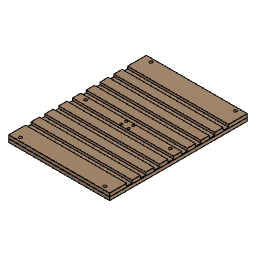
X platform (Autodesk Fusion 360 design; units mm, degrees)
Autodesk Fusion 360 part; units mm, degrees
sketch "Bottom" plane through (0, 0, 0) normal (0, 0, 1) x (1, 0, 0)
  line L0 (275, 375) -> (-275, 375)
  line L1 (-275, 375) -> (-275, -375)
  line L2 (-275, -375) -> (275, -375)
  line L3 (275, -375) -> (275, 375)
  line L4 (275, 375) -> (-275, -375) construction
  line L5 (-275, 375) -> (275, -375) construction
  line L6 (155, 375) -> (155, -375) construction
  line L7 (-155, 375) -> (-155, -375) construction
  line L8 (-155, 349.39) -> (-140, 349.39) construction
  line L9 (-140, 349.39) -> (-140, -349.39) construction
  line L10 (-140, -349.39) -> (-170, -349.39) construction
  line L11 (-170, -349.39) -> (-170, 349.39) construction
  line L12 (-170, 349.39) -> (-155, 349.39) construction
  line L13 (155, 350.2785) -> (170, 350.2785) construction
  line L14 (170, 350.2785) -> (170, -350.2785) construction
  line L15 (170, -350.2785) -> (140, -350.2785) construction
  line L16 (140, -350.2785) -> (140, 350.2785) construction
  line L17 (140, 350.2785) -> (155, 350.2785) construction
  line L18 (-170, 0) -> (170, 0) construction
  line L19 (-170, 300) -> (170, 300) construction
  line L20 (-170, 150) -> (170, 150) construction
  line L21 (-170, -150) -> (170, -150) construction
  line L22 (-170, -300) -> (170, -300) construction
  circle A0 centre (-170, -300) radius 3
  circle A1 centre (-140, -300) radius 3
  circle A2 centre (140, -300) radius 3
  circle A3 centre (170, -300) radius 3
  circle A4 centre (-170, -150) radius 3
  circle A5 centre (-140, -150) radius 3
  circle A6 centre (140, -150) radius 3
  circle A7 centre (170, -150) radius 3
  circle A8 centre (-170, 0) radius 3
  circle A9 centre (-140, 0) radius 3
  circle A10 centre (140, 0) radius 3
  circle A11 centre (170, 0) radius 3
  circle A12 centre (-170, 150) radius 3
  circle A13 centre (-140, 150) radius 3
  circle A14 centre (140, 150) radius 3
  circle A15 centre (170, 150) radius 3
  circle A16 centre (-170, 300) radius 3
  circle A17 centre (-140, 300) radius 3
  circle A18 centre (140, 300) radius 3
  circle A19 centre (170, 300) radius 3
  line L23 (-18.5, 7) -> (21.5, 7) construction
  line L24 (21.5, 7) -> (21.5, -17) construction
  line L25 (21.5, -17) -> (-18.5, -17) construction
  line L26 (-18.5, -17) -> (-18.5, 7) construction
  circle A20 centre (-18.5, 7) radius 3
  circle A21 centre (21.5, 7) radius 3
  circle A22 centre (21.5, -17) radius 3
  circle A23 centre (-18.5, -17) radius 3
  circle A24 centre (-230, 355) radius 3.5
  circle A25 centre (-230, 355) radius 7.95
  circle A26 centre (230, 355) radius 3.5
  circle A27 centre (230, 355) radius 7.95
  circle A28 centre (230, -355) radius 3.5
  circle A29 centre (230, -355) radius 7.95
  circle A30 centre (-230, -355) radius 3.5
  circle A31 centre (-230, -355) radius 7.95
  circle A32 centre (-170, 300) radius 6.35
  circle A33 centre (-140, 300) radius 6.35
  circle A34 centre (-170, 150) radius 6.35
  circle A35 centre (-140, 150) radius 6.35
  circle A36 centre (-170, 0) radius 6.35
  circle A37 centre (-140, 0) radius 6.35
  circle A38 centre (-170, -150) radius 6.35
  circle A39 centre (-140, -150) radius 6.35
  circle A40 centre (-170, -300) radius 6.35
  circle A41 centre (-140, -300) radius 6.35
  circle A42 centre (140, -300) radius 6.35
  circle A43 centre (170, -300) radius 6.35
  circle A44 centre (140, -150) radius 6.35
  circle A45 centre (170, -150) radius 6.35
  circle A46 centre (140, 0) radius 6.35
  circle A47 centre (170, 0) radius 6.35
  circle A48 centre (140, 150) radius 6.35
  circle A49 centre (170, 150) radius 6.35
  circle A50 centre (140, 300) radius 6.35
  circle A51 centre (170, 300) radius 6.35
  circle A52 centre (-18.5, 7) radius 6.35
  circle A53 centre (21.5, 7) radius 6.35
  circle A54 centre (-18.5, -17) radius 6.35
  circle A55 centre (21.5, -17) radius 6.35
  line L27 (230, -355) -> (230, 355) construction
  line L28 (-230, 355) -> (-230, -355) construction
  circle A56 centre (230, 0) radius 3.5
  circle A57 centre (230, 0) radius 7.95
  circle A58 centre (-230, 0) radius 3.5
  circle A59 centre (-230, 0) radius 7.95
  dimension "d1" = 550
  dimension "d2" = 750
  dimension "d3" = 120
  dimension "d4" = 310
  dimension "d5" = 120
  dimension "d6" = 30
  dimension "d7" = 30
  dimension "d9" = 150
  dimension "d10" = 150
  dimension "d11" = 150
  dimension "d12" = 150
  dimension "d13" = 6
  dimension "d14" = 6
  dimension "d15" = 6
  dimension "d16" = 6
  dimension "d17" = 6
  dimension "d18" = 6
  dimension "d19" = 6
  dimension "d20" = 6
  dimension "d21" = 6
  dimension "d22" = 6
  dimension "d23" = 6
  dimension "d24" = 6
  dimension "d25" = 6
  dimension "d26" = 6
  dimension "d27" = 6
  dimension "d28" = 6
  dimension "d29" = 6
  dimension "d30" = 6
  dimension "d31" = 6
  dimension "d32" = 6
  dimension "d33" = 75
  dimension "d36" = 24
  dimension "d37" = 368
  dimension "d38" = 358
  dimension "d39" = 253.5
  dimension "d40" = 256.5
  dimension "d41" = 40
  dimension "d42" = 6
  dimension "d43" = 6
  dimension "d44" = 6
  dimension "d45" = 6
  dimension "d46" = 7
  dimension "d47" = 15.9
  dimension "d48" = 20
  dimension "d49" = 45
  dimension "d50" = 7
  dimension "d51" = 15.9
  dimension "d52" = 45
  dimension "d53" = 20
  dimension "d54" = 7
  dimension "d55" = 15.9
  dimension "d56" = 45
  dimension "d57" = 20
  dimension "d58" = 7
  dimension "d59" = 15.9
  dimension "d60" = 20
  dimension "d61" = 45
  dimension "d74" = 12.7
  dimension "d75" = 12.7
  dimension "d76" = 12.7
  dimension "d77" = 12.7
  dimension "d78" = 12.7
  dimension "d79" = 12.7
  dimension "d80" = 12.7
  dimension "d81" = 12.7
  dimension "d82" = 12.7
  dimension "d83" = 12.7
  dimension "d84" = 12.7
  dimension "d85" = 12.7
  dimension "d86" = 12.7
  dimension "d87" = 12.7
  dimension "d88" = 12.7
  dimension "d89" = 12.7
  dimension "d90" = 12.7
  dimension "d91" = 12.7
  dimension "d92" = 12.7
  dimension "d93" = 12.7
  dimension "d122" = 12.7
  dimension "d123" = 12.7
  dimension "d124" = 12.7
  dimension "d125" = 12.7
  dimension "d167" = 7
  dimension "d168" = 15.9
  dimension "d169" = 7
  dimension "d170" = 15.9
  constraint perpendicular L0 L1
  constraint parallel L0 L2
  constraint parallel L1 L3
  constraint horizontal L0
  constraint coincident L4 origin
  constraint coincident L5 origin
  constraint coincident L0 L6.start
  constraint perpendicular L0 L6
  constraint coincident L0 L7.start
  constraint coincident L2 L7.end
  constraint perpendicular L2 L7
  constraint coincident L7 L8.start
  constraint perpendicular L7 L8
  constraint perpendicular L8 L9
  constraint perpendicular L7 L10
  constraint perpendicular L10 L11
  constraint collinear L8 L12
  constraint equal L8 L12
  constraint coincident L6 L13.start
  constraint perpendicular L6 L13
  constraint perpendicular L13 L14
  constraint perpendicular L6 L15
  constraint perpendicular L15 L16
  constraint perpendicular L6 L17
  constraint equal L13 L17
  constraint midpoint L11 L18.start
  constraint midpoint L14 L18.end
  constraint coincident L11 L19.start
  constraint coincident L14 L19.end
  constraint perpendicular L14 L19
  constraint perpendicular L9 L18
  constraint coincident L11 L20.start
  constraint coincident L14 L20.end
  constraint perpendicular L14 L20
  constraint coincident L11 L21.start
  constraint coincident L14 L21.end
  constraint perpendicular L14 L21
  constraint coincident L11 L22.start
  constraint coincident L14 L22.end
  constraint perpendicular L14 L22
  constraint coincident L22.start A0.centre
  constraint coincident L9 A1.centre
  constraint coincident L22 A1.centre
  constraint coincident L16 A2.centre
  constraint coincident L22 A2.centre
  constraint coincident L22.end A3.centre
  constraint coincident L21.start A4.centre
  constraint coincident L9 A5.centre
  constraint coincident L21 A5.centre
  constraint coincident L16 A6.centre
  constraint coincident L21 A6.centre
  constraint coincident L21.end A7.centre
  constraint coincident L18.start A8.centre
  constraint midpoint L9 A9.centre
  constraint midpoint L16 A10.centre
  constraint coincident L18.end A11.centre
  constraint coincident L20.start A12.centre
  constraint coincident L9 A13.centre
  constraint coincident L20 A13.centre
  constraint coincident L16 A14.centre
  constraint coincident L20 A14.centre
  constraint coincident L20.end A15.centre
  constraint coincident L19.start A16.centre
  constraint coincident L19 A17.centre
  constraint coincident L9 A17.centre
  constraint coincident L16 A18.centre
  constraint coincident L19 A18.centre
  constraint coincident L19.end A19.centre
  constraint horizontal L23
  constraint vertical L24
  constraint horizontal L25
  constraint vertical L26
  constraint coincident L23.start L26.end
  constraint coincident L23.end L24.start
  constraint coincident L24.end L25.start
  constraint coincident L25.end L26.start
  constraint concentric A24 A25
  constraint concentric A26 A27
  constraint concentric A28 A29
  constraint concentric A30 A31
  constraint concentric A16 A32
  constraint concentric A17 A33
  constraint concentric A12 A34
  constraint concentric A13 A35
  constraint concentric A8 A36
  constraint concentric A9 A37
  constraint concentric A4 A38
  constraint concentric A5 A39
  constraint concentric A0 A40
  constraint concentric A1 A41
  constraint concentric A2 A42
  constraint concentric A3 A43
  constraint concentric A6 A44
  constraint concentric A7 A45
  constraint concentric A10 A46
  constraint concentric A11 A47
  constraint concentric A14 A48
  constraint concentric A15 A49
  constraint concentric A18 A50
  constraint concentric A19 A51
  constraint concentric A20 A52
  constraint concentric A21 A53
  constraint concentric A23 A54
  constraint concentric A22 A55
  constraint coincident A28.centre A29.centre
  constraint coincident A26.centre A27.centre
  constraint coincident A24.centre A25.centre
  constraint coincident A30.centre A31.centre
  constraint midpoint L27 A56.centre
  constraint concentric A56 A57
  constraint midpoint L28 A58.centre
  constraint concentric A58 A59
  measures "d1" distance of L1.end L2.end
  measures "d2" distance of L0.end L1.end
  measures "d3" distance of L3 L6
  measures "d4" distance of L6 L7
  measures "d5" distance of L1 L7
  measures "d6" distance of L9 L11
  measures "d7" distance of L14 L16
  measures "d9" distance of L18 L20
  measures "d10" distance of L19 L20
  measures "d11" distance of L18 L21
  measures "d12" distance of L21 L22
  measures "d13" diameter of A0
  measures "d14" diameter of A1
  measures "d15" diameter of A2
  measures "d16" diameter of A3
  measures "d17" diameter of A4
  measures "d18" diameter of A5
  measures "d19" diameter of A6
  measures "d20" diameter of A7
  measures "d21" diameter of A8
  measures "d22" diameter of A9
  measures "d23" diameter of A10
  measures "d24" diameter of A11
  measures "d25" diameter of A12
  measures "d26" diameter of A13
  measures "d27" diameter of A14
  measures "d28" diameter of A15
  measures "d29" diameter of A16
  measures "d30" diameter of A17
  measures "d31" diameter of A18
  measures "d32" diameter of A19
  measures "d33" distance of L0 L19
  measures "d36" distance of L23.start L25.end
  measures "d37" distance of L0 L23
  measures "d38" distance of L2 L25
  measures "d39" distance of L3 L24
  measures "d40" distance of L1 L26
  measures "d41" distance of L24 L26
  measures "d42" diameter of A20
  measures "d43" diameter of A21
  measures "d44" diameter of A22
  measures "d45" diameter of A23
  measures "d46" diameter of A24
  measures "d47" diameter of A25
  measures "d48" distance of L0 A24.centre
  measures "d49" distance of L1 A24.centre
  measures "d50" diameter of A26
  measures "d51" diameter of A27
  measures "d52" distance of L3 A26.centre
  measures "d53" distance of L0 A26.centre
  measures "d54" diameter of A28
  measures "d55" diameter of A29
  measures "d56" distance of L3 A28.centre
  measures "d57" distance of L2 A28.centre
  measures "d58" diameter of A30
  measures "d59" diameter of A31
  measures "d60" distance of L2 A30.centre
  measures "d61" distance of L1 A30.centre
  measures "d74" diameter of A32
  measures "d75" diameter of A33
  measures "d76" diameter of A34
  measures "d77" diameter of A35
  measures "d78" diameter of A36
  measures "d79" diameter of A37
  measures "d80" diameter of A38
  measures "d81" diameter of A39
  measures "d82" diameter of A40
  measures "d83" diameter of A41
  measures "d84" diameter of A42
  measures "d85" diameter of A43
  measures "d86" diameter of A44
  measures "d87" diameter of A45
  measures "d88" diameter of A46
  measures "d89" diameter of A47
  measures "d90" diameter of A48
  measures "d91" diameter of A49
  measures "d92" diameter of A50
  measures "d93" diameter of A51
  measures "d122" diameter of A52
  measures "d123" diameter of A53
  measures "d124" diameter of A54 L0.start
  measures "d125" diameter of A55
  measures "d167" diameter of A56
  measures "d168" diameter of A57
  measures "d169" diameter of A58
  measures "d170" diameter of A59
extrude "Extrude24" add sketch "Bottom" against normal blind 18 contours L0 L1 L2 L3 | A25 | A27 | A29 | A31 | A32 | A33 | A34 | A35 | A36 | A37 | A38 | A39 | A40 | A41 | A42 | A43 | A44 | A45 | A46 | A47 | A48 | A49 | A50 | A51 | A52 | A53 | A54 | A55 | A57 | A59 makes body 1
extrude "Extrude27" cut sketch "Bottom" against normal through all from surface at -9 contours A25 | A27 | A29 | A31 | A57 | A59 bodies 1
extrude "Extrude28" cut sketch "Bottom" against normal blind 8 contours A32 | A33 | A34 | A35 | A36 | A37 | A38 | A39 | A40 | A41 | A42 | A43 | A44 | A45 | A46 | A47 | A48 | A49 | A50 | A51 bodies 1
fillet "Fillet1" radius 0.5 12 edges at (-275, 0, 0) (-275, 0, -18) (0, -375, 0) (0, -375, -18) (275, 0, 0) (275, 0, -18) (0, 375, 0) (0, 375, -18) (-275, 375, -9) (-275, -375, -9) (275, -375, -9) (275, 375, -9) on bodies 1
extrude "Extrude25" add sketch "Bottom" along normal blind 8 separate body contours A25 | A27 | A29 | A31 | A57 | A59 makes body 2 at (237.7042, -353.0383, 5.3333) makes body 3 at (-222.2958, 356.9617, 5.3333) makes body 4 at (-222.2958, -353.0383, 5.3333) makes body 5 at (237.7042, 356.9617, 5.3333) makes body 6 at (-222.0599, -0.3963, 5.3333) makes body 7 at (237.9401, -0.3963, 5.3333)
extrude "Extrude26" add sketch "Bottom" along normal blind 18 contours L0 L1 L2 L3 | A0 | A1 | A2 | A3 | A4 | A5 | A6 | A7 | A8 | A9 | A10 | A11 | A12 | A13 | A14 | A15 | A16 | A17 | A18 | A19 | A32 | A33 | A34 | A35 | A36 | A37 | A38 | A39 | A40 | A41 | A42 | A43 | A44 | A45 | A46 | A47 | A48 | A49 | A50 | A51 bodies 6 3 7 2 5 4
extrude "Extrude29" cut sketch "Bottom" along normal blind 8 contours A0 | A1 | A2 | A3 | A4 | A5 | A6 | A7 | A8 | A9 | A10 | A11 | A12 | A13 | A14 | A15 | A16 | A17 | A18 | A19 | A20 | A21 | A22 | A23 | A32 | A33 | A34 | A35 | A36 | A37 | A38 | A39 | A40 | A41 | A42 | A43 | A44 | A45 | A46 | A47 | A48 | A49 | A50 | A51 | A52 | A53 | A54 | A55 bodies 6
fillet "Fillet3" radius 0.5 12 edges at (0, 375, 18) (0, 375, 0) (-275, 375, 9) (-275, 0, 18) (-275, 0, 0) (-275, -375, 9) (0, -375, 18) (0, -375, 0) (275, 375, 9) (275, 0, 18) (275, 0, 0) (275, -375, 9) on bodies 6
sketch "Side" plane through (275, 0, 0) normal (1, 0, 0) x (0, 1, 0)
  line L0 (-375, 0) -> (375, 0)
  line L1 (375, 0) -> (375, 25)
  line L2 (375, 25) -> (-375, 25)
  line L3 (-375, 25) -> (-375, 0)
  line L4 (-391.2499, 11.5) -> (399.4526, 11.5) construction
  line L5 (399.4526, 11.5) -> (389.4526, 11.5) construction
  line L6 (-27.5, 18) -> (-57.5, 18)
  line L7 (-57.5, 18) -> (-57.5, 5)
  line L8 (-57.5, 5) -> (-27.5, 5)
  line L9 (-27.5, 5) -> (-27.5, 18)
  line L10 (-27.5, 18) -> (-57.5, 5) construction
  line L11 (-57.5, 18) -> (-27.5, 5) construction
  line L12 (-102.5, 18) -> (-132.5, 18)
  line L13 (-132.5, 18) -> (-132.5, 5)
  line L14 (-132.5, 5) -> (-102.5, 5)
  line L15 (-102.5, 5) -> (-102.5, 18)
  line L16 (-102.5, 18) -> (-132.5, 5) construction
  line L17 (-132.5, 18) -> (-102.5, 5) construction
  line L18 (47.5, 18) -> (17.5, 18)
  line L19 (17.5, 18) -> (17.5, 5)
  line L20 (17.5, 5) -> (47.5, 5)
  line L21 (47.5, 5) -> (47.5, 18)
  line L22 (47.5, 18) -> (17.5, 5) construction
  line L23 (17.5, 18) -> (47.5, 5) construction
  line L24 (122.5, 18) -> (92.5, 18)
  line L25 (92.5, 18) -> (92.5, 5)
  line L26 (92.5, 5) -> (122.5, 5)
  line L27 (122.5, 5) -> (122.5, 18)
  line L28 (122.5, 18) -> (92.5, 5) construction
  line L29 (92.5, 18) -> (122.5, 5) construction
  line L30 (197.5, 18) -> (167.5, 18)
  line L31 (167.5, 18) -> (167.5, 5)
  line L32 (167.5, 5) -> (197.5, 5)
  line L33 (197.5, 5) -> (197.5, 18)
  line L34 (197.5, 18) -> (167.5, 5) construction
  line L35 (167.5, 18) -> (197.5, 5) construction
  line L36 (-177.5, 18) -> (-207.5, 18)
  line L37 (-207.5, 18) -> (-207.5, 5)
  line L38 (-207.5, 5) -> (-177.5, 5)
  line L39 (-177.5, 5) -> (-177.5, 18)
  line L40 (-177.5, 18) -> (-207.5, 5) construction
  line L41 (-207.5, 18) -> (-177.5, 5) construction
  line L42 (272.5, 18) -> (242.5, 18)
  line L43 (242.5, 18) -> (242.5, 5)
  line L44 (242.5, 5) -> (272.5, 5)
  line L45 (272.5, 5) -> (272.5, 18)
  line L46 (272.5, 18) -> (242.5, 5) construction
  line L47 (242.5, 18) -> (272.5, 5) construction
  line L48 (-252.5, 18) -> (-282.5, 18)
  line L49 (-282.5, 18) -> (-282.5, 5)
  line L50 (-282.5, 5) -> (-252.5, 5)
  line L51 (-252.5, 5) -> (-252.5, 18)
  line L52 (-252.5, 18) -> (-282.5, 5) construction
  line L53 (-282.5, 18) -> (-252.5, 5) construction
  line L54 (-375, 0) -> (375, 0)
  line L55 (-374.5, 17.5) -> (-374.5, 0.5)
  line L56 (-374.5, 0.5) -> (374.5, 0.5)
  line L57 (374.5, 0.5) -> (374.5, 17.5)
  line L58 (374.5, 17.5) -> (-374.5, 17.5)
  point P0 (-42.5, 11.5)
  point P1 (-117.5, 11.5)
  point P2 (32.5, 11.5)
  point P3 (107.5, 11.5)
  point P4 (182.5, 11.5)
  point P5 (-192.5, 11.5)
  point P6 (257.5, 11.5)
  point P7 (-267.5, 11.5)
  dimension "d131" = 30
  dimension "d132" = 30
  dimension "d133" = 30
  dimension "d134" = 30
  dimension "d135" = 30
  dimension "d136" = 30
  dimension "d137" = 75
  dimension "d138" = 75
  dimension "d139" = 75
  dimension "d140" = 75
  dimension "d141" = 75
  dimension "d142" = 32.5
  dimension "d143" = 30
  dimension "d144" = 30
  dimension "d145" = 75
  dimension "d146" = 75
  dimension "d154" = 11.5
  dimension "d155" = 13
  dimension "d156" = 13
  dimension "d157" = 13
  dimension "d158" = 13
  dimension "d159" = 13
  dimension "d160" = 13
  dimension "d161" = 13
  dimension "d162" = 13
  constraint perpendicular L1 L4
  constraint coincident L4 L5.end
  constraint perpendicular L6 L7
  constraint parallel L6 L8
  constraint parallel L7 L9
  constraint horizontal L6
  constraint coincident L10 P0
  constraint coincident L11 P0
  constraint coincident L4 P0
  constraint perpendicular L12 L13
  constraint parallel L12 L14
  constraint parallel L13 L15
  constraint horizontal L12
  constraint coincident L16 P1
  constraint coincident L17 P1
  constraint coincident L4 P1
  constraint perpendicular L18 L19
  constraint parallel L18 L20
  constraint parallel L19 L21
  constraint horizontal L18
  constraint coincident L22 P2
  constraint coincident L23 P2
  constraint coincident L4 P2
  constraint perpendicular L24 L25
  constraint parallel L24 L26
  constraint parallel L25 L27
  constraint horizontal L24
  constraint coincident L28 P3
  constraint coincident L29 P3
  constraint coincident L4 P3
  constraint perpendicular L30 L31
  constraint parallel L30 L32
  constraint parallel L31 L33
  constraint horizontal L30
  constraint coincident L34 P4
  constraint coincident L35 P4
  constraint coincident L4 P4
  constraint perpendicular L36 L37
  constraint parallel L36 L38
  constraint parallel L37 L39
  constraint horizontal L36
  constraint coincident L40 P5
  constraint coincident L41 P5
  constraint coincident L4 P5
  constraint perpendicular L42 L43
  constraint parallel L42 L44
  constraint parallel L43 L45
  constraint horizontal L42
  constraint coincident L46 P6
  constraint coincident L47 P6
  constraint coincident L4 P6
  constraint perpendicular L48 L49
  constraint parallel L48 L50
  constraint parallel L49 L51
  constraint horizontal L48
  constraint coincident L52 P7
  constraint coincident L53 P7
  constraint coincident L4 P7
  measures "d131" distance of L7.end L8.end
  measures "d132" distance of L13.end L14.end
  measures "d133" distance of L19.end L20.end
  measures "d134" distance of L25.end L26.end
  measures "d135" distance of L31.end L32.end
  measures "d136" distance of L37.end L38.end
  measures "d137" distance of P0 P2
  measures "d138" distance of P2 P3
  measures "d139" distance of P3 P4
  measures "d140" distance of P0 P1
  measures "d141" distance of P1 P5
  measures "d142" horizontal distance of origin P2
  measures "d143" distance of L43.end L44.end
  measures "d144" distance of L49.end L50.end
  measures "d145" distance of P5 P7
  measures "d146" distance of P4 P6
  measures "d154" distance of L4 L54
  measures "d156" distance of L18.end L19.end
  measures "d157" distance of L24.end L25.end
  measures "d158" distance of L30.end L31.end
  measures "d159" distance of L42.end L43.end
  measures "d160" distance of L12.end L13.end
  measures "d161" distance of L36.end L37.end
  measures "d162" distance of L48.end L49.end
extrude "Extrude23" cut sketch "Side" against normal through all contours L6 L7 L9 L58 | L7 L8 L9 L58 | L19 L20 L21 L58 | L18 L19 L21 L58 | L12 L13 L15 L58 | L13 L14 L15 L58 | L25 L26 L27 L58 | L24 L25 L27 L58 | L36 L37 L39 L58 | L37 L38 L39 L58 | L31 L32 L33 L58 | L30 L31 L33 L58 | L48 L49 L51 L58 | L49 L50 L51 L58 | L43 L44 L45 L58 | L42 L43 L45 L58 bodies 6
equation "d13 = d29"
equation "d14 = d29"
equation "d15 = d29"
equation "d16 = d29"
equation "d17 = d29"
equation "d18 = d29"
equation "d19 = d29"
equation "d20 = d29"
equation "d21 = d29"
equation "d22 = d29"
equation "d23 = d29"
equation "d24 = d29"
equation "d25 = d29"
equation "d26 = d29"
equation "d27 = d29"
equation "d28 = d29"
equation "d30 = d29"
equation "d31 = d29"
equation "d32 = d29"
equation "d43 = d42"
equation "d44 = d42"
equation "d45 = d42"
equation "d50 = d46"
equation "d51 = d47"
equation "d54 = d46"
equation "d55 = d47"
equation "d58 = d46"
equation "d59 = d47"
equation "d74 = d122"
equation "d75 = d122"
equation "d76 = d122"
equation "d77 = d122"
equation "d78 = d122"
equation "d79 = d122"
equation "d80 = d122"
equation "d81 = d122"
equation "d82 = d122"
equation "d83 = d122"
equation "d84 = d122"
equation "d85 = d122"
equation "d86 = d122"
equation "d87 = d122"
equation "d88 = d122"
equation "d89 = d122"
equation "d90 = d122"
equation "d91 = d122"
equation "d92 = d122"
equation "d93 = d122"
equation "d123 = d122"
equation "d124 = d122"
equation "d125 = d122"
equation "d138 = d137"
equation "d139 = d137"
equation "d140 = d137"
equation "d141 = d137"
equation "d145 = d137"
equation "d146 = d137"
equation "d154 = 18 mm - d155 / 2"
equation "d156 = d155"
equation "d157 = d155"
equation "d158 = d155"
equation "d159 = d155"
equation "d160 = d155"
equation "d161 = d155"
equation "d162 = d155"
equation "d167 = d46"
equation "d168 = d47"
equation "d169 = d46"
equation "d170 = d47"
named bodies: "LowerPlatform", "UpperPlatform"
